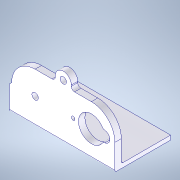
# Autodesk Inventor part: sheet4
Saved by Autodesk Inventor 2022 (Build 260153000, 153)
## iProperties
Created: 2016-01-20
Part Number: sheet4
Material: ABS Plastic
Document SubType Name: Modeling
Designer: Nanjar
Density: 1.06 g/cm^3
Appearance: Cool White
Author: Nanjar
Autodesk Inventor part; units mm, degrees
ref_plane "YZ Plane" through (0, 0, 0) normal (1, 0, 0) x (0, 1, 0)
ref_plane "XZ Plane" through (0, 0, 0) normal (0, 1, 0) x (-1, 0, 0)
ref_plane "XY Plane" through (0, 0, 0) normal (0, 0, 1) x (1, 0, 0)
sketch "Sketch1" plane through (0, 0, 0) normal (0, 0, 1) x (1, 0, 0)
  arc A0 (-26.3575, 9.02) -> (-37.2975, -1.92) centre (-26.3575, -1.92) ccw
  line L0 (-37.2975, -1.92) -> (-38.3625, -2.985)
  arc A1 (10.8425, -1.92) -> (-0.0975, 9.02) centre (-0.0975, -1.92) ccw
  circle A2 centre (-13.2275, 11.07) radius 1.5
  arc A3 (-9.4775, 11.07) -> (-16.9775, 11.07) centre (-13.2275, 11.07) ccw
  line L1 (-16.9775, 11.07) -> (-16.9775, 9.02)
  line L2 (-9.4775, 11.07) -> (-9.4775, 9.02)
  line L3 (-26.3575, 9.02) -> (-16.9775, 9.02)
  line L4 (-9.4775, 9.02) -> (-0.0975, 9.02)
  line L5 (10.8425, -1.92) -> (10.8425, -15)
  line L6 (-38.3625, -15) -> (10.8425, -15)
  circle A4 centre (-26.3575, -1.92) radius 1.5
  arc A5 (5.4151, 0.5728) -> (5.4151, -4.4128) centre (-0.0975, -1.92) ccw
  arc A6 (6.337, -4.4408) -> (6.337, 0.6008) centre (5.9521, -1.92) ccw
  arc A7 (5.4151, -4.4128) -> (5.4151, 0.5728) centre (5.9521, -1.92) ccw
  line L7 (-38.3625, -2.985) -> (-38.3625, -15)
  dimension "d0" = 3
  dimension "d1" = 7.5
  constraints: 16 end point, 12 point on circle, 8 centre point, 6 coincident, 3 vertical, 2 perpendicular, 2 tangent
  measures "d0" diameter of A2
  measures "d1" diameter of A3
extrude "Extrusion1" add sketch "Sketch1" along normal blind 3
fillet "Fillet1" radius 1.5 2 edges at (-9.4775, 9.02, 1.5) (-16.9775, 9.02, 1.5)
fillet "Fillet2" radius 1.5 2 edges at (5.4151, 0.5728, 1.5) (5.4151, -4.4128, 1.5)
sketch "Sketch2" plane through (0, 0, 0) normal (0, 0, -1) x (-1, 0, 0)
  line L0 (-7.8651, -12) -> (38.3625, -12)
  line L1 (38.3625, -12) -> (38.3625, -15)
  line L2 (38.3625, -12) -> (-10.8425, -12)
  line L3 (-10.8425, -12) -> (-10.8425, -15)
  line L4 (38.3625, -15) -> (-10.8425, -15)
  constraints: 10 end point, 2 horizontal, 1 perpendicular
extrude "Extrusion2" add sketch "Sketch2" along normal blind 23
fillet "Fillet3" radius 0.8 2 edges at (-13.76, -12, 0) (-13.76, -15, 3)
sketch "Sketch5" plane through (0, 0, 0) normal (0, 0, -1) x (-1, 0, 0)
  circle A0 centre (8.5925, -1.92) radius 0.85
  line L0 (-10.8425, -15) -> (38.3625, -15) projected
  line L1 (38.3625, -2.985) -> (38.3625, -11.2) projected
  point P0 (0, 0)
  point P1 (6.3625, -15)
  dimension "d20" = 1.7
  dimension "d21" = 13.08
  dimension "d22" = 29.77
  constraints: 1 centre point
  measures "d20" diameter of A0
  measures "d21" distance from line of L0 A0.centre
  measures "d22" distance from line of L1 A0.centre
extrude "Extrusion5" cut sketch "Sketch5" against normal through all
move faces "Move3" translate (0, 1, 0) faces at (-5.5592, -15, -6.2)
sketch "Sketch10" plane through (-38.3625, -14, 2.2) normal (0, -1, 0) x (1, 0, 0)
  line L0 (0, -25.2) -> (0, 0) projected
  line L1 (0, 0) -> (49.205, 0) projected
  circle A0 centre (24.6025, -12.6) radius 0.05
  point P0 (38.3625, -2.2)
  dimension "d47" = 0.1
  constraints: 1 centre point, 1 coincident
  measures "d47" diameter of A0
extrude "Extrusion8" cut sketch "Sketch10" against normal blind 1
body "Solid1"
